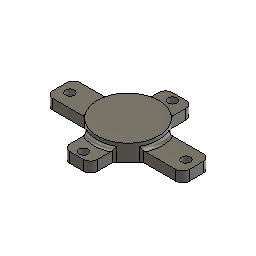
Base (Autodesk Fusion 360 design; units mm, degrees)
part number: 2025-04-16-17-35-49-953
Autodesk Fusion 360 part; units mm, degrees
sketch "Sketch1" plane through (0, 0, 0) normal (0, 1, 0) x (1, 0, 0)
  line L0 (20, 75) -> (-20, 75)
  line L1 (-100, 20) -> (-100, -20)
  line L2 (-20, -75) -> (20, -75)
  line L3 (100, -20) -> (100, 20)
  line L4 (20, 40.3113) -> (20, 75)
  line L5 (20, 75) -> (-20, 75)
  line L6 (-20, 75) -> (-20, 40.3113)
  line L7 (20, -40.3113) -> (20, -75)
  line L8 (20, -75) -> (-20, -75)
  line L9 (-20, -75) -> (-20, -40.3113)
  line L10 (40.3113, 20) -> (100, 20)
  line L11 (100, 20) -> (100, -20)
  line L12 (100, -20) -> (40.3113, -20)
  line L13 (-40.3113, 20) -> (-100, 20)
  line L14 (-100, 20) -> (-100, -20)
  line L15 (-100, -20) -> (-30, -20)
  arc A0 (-20, 40.3113) -> (-40.3113, 20) centre (0, 0) ccw
  arc A1 (40.3113, 20) -> (20, 40.3113) centre (0, 0) ccw
  arc A2 (-40.3113, -20) -> (-20, -40.3113) centre (0, 0) ccw
  arc A3 (20, -40.3113) -> (40.3113, -20) centre (0, 0) ccw
  dimension "d5" = 90
  constraint horizontal L0
  constraint perpendicular L0 L1
  constraint parallel L0 L2
  constraint parallel L1 L3
  constraint coincident A0.centre A1.centre
  constraint vertical L4
  constraint horizontal L5
  constraint vertical L6
  constraint vertical L7
  constraint horizontal L8
  constraint vertical L9
  constraint horizontal L10
  constraint vertical L11
  constraint horizontal L12
  constraint horizontal L13
  constraint vertical L14
  constraint horizontal L15
  constraint coincident L9.end A0
  constraint coincident L15 A2.start
  constraint concentric A0 A2
  constraint concentric A1 A2
  constraint coincident L7.start A2
  constraint concentric A2 A3
  measures "d5" diameter of A0
extrude "Extrude1" add sketch "Sketch1" along normal blind 15
sketch "Sketch3" plane through (0, 15, 0) normal (0, 1, 0) x (-1, 0, 0)
  line L0 (-20, 75) -> (-20, 40.3113)
  arc A0 (-20, 40.3113) -> (-40.3113, 20) centre (0, 0) ccw
  line L1 (-40.3113, 20) -> (-100, 20)
  line L2 (-100, 20) -> (-100, -20)
  line L3 (-100, -20) -> (-40.3113, -20)
  arc A1 (-40.3113, -20) -> (-20, -40.3113) centre (0, 0) ccw
  line L4 (-20, -40.3113) -> (-20, -75)
  line L5 (-20, -75) -> (20, -75)
  line L6 (20, -75) -> (20, -40.3113)
  arc A2 (20, -40.3113) -> (40.3113, -20) centre (0, 0) ccw
  line L7 (40.3113, -20) -> (100, -20)
  line L8 (100, -20) -> (100, 20)
  line L9 (100, 20) -> (40.3113, 20)
  arc A3 (40.3113, 20) -> (20, 40.3113) centre (0, 0) ccw
  line L10 (20, 40.3113) -> (20, 75)
  line L11 (20, 75) -> (-20, 75)
  circle A4 centre (0, 0) radius 45
  constraint coincident A0.centre A1.centre
extrude "Extrude2" add sketch "Sketch3" along normal blind 10 contours A0 A1 A2 A3 A4
fillet "Fillet1" radius 5 1 edges at (0, 15, 45)
fillet "Fillet2" radius 5 1 edges at (45, 15, 0)
fillet "Fillet3" radius 5 1 edges at (0, 15, -45)
fillet "Fillet4" radius 5 1 edges at (-45, 15, 0)
fillet "Fillet5" radius 5 1 edges at (-20, 10, -40.3113)
fillet "Fillet6" radius 5 1 edges at (-40.3113, 10, -20)
fillet "Fillet7" radius 5 1 edges at (-40.3113, 10, 20)
fillet "Fillet8" radius 5 1 edges at (-20, 10, 40.3113)
fillet "Fillet9" radius 5 1 edges at (20, 10, 40.3113)
fillet "Fillet10" radius 5 1 edges at (40.3113, 10, 20)
sketch "Sketch4" plane through (0, 15, 0) normal (0, 1, 0) x (-1, 0, 0)
  arc A0 (45.8258, -20) -> (45.8258, 20) centre (0, 0) ccw
  line L0 (45.8258, -20) -> (100, -20)
  line L1 (100, -20) -> (100, 20)
  line L2 (100, 20) -> (45.8258, 20)
  circle A1 centre (0, -65) radius 6.5
  circle A2 centre (0, 65) radius 6.5
  circle A3 centre (-85, 0) radius 6.5
  circle A4 centre (85, 0) radius 6.5
  dimension "d30" = 13
  dimension "d31" = 13
  dimension "d32" = 13
  dimension "d33" = 13
  measures "d30" diameter of A1
  measures "d31" diameter of A2
  measures "d32" diameter of A3
  measures "d33" diameter of A4
extrude "Extrude3" cut sketch "Sketch4" against normal blind 15 contours A1 | A2 | A3 | A4
fillet "Fillet11" radius 10 1 edges at (20, 7.5, 75)
fillet "Fillet12" radius 10 7 edges at (100, 7.5, 20) (100, 7.5, -20) (20, 7.5, -75) (-100, 7.5, 20) (-20, 7.5, 75) (-20, 7.5, -75) (-100, 7.5, -20)
sketch "Sketch5" plane through (0, 0, 0) normal (0, -1, 0) x (1, 0, 0)
  circle A0 centre (0, -65) radius 6.5
  circle A1 centre (85, 0) radius 6.5
  circle A2 centre (-85, 0) radius 6.5
  circle A3 centre (0, 65) radius 6.5
  arc A4 (-100, -10) -> (-90, -20) centre (-90, -10) ccw
  line L0 (-90, -20) -> (-43.3013, -20)
  arc A5 (-38.9711, -22.5) -> (-43.3013, -20) centre (-43.3013, -25) ccw
  arc A6 (-38.9711, -22.5) -> (-22.5, -38.9711) centre (0, 0) ccw
  arc A7 (-20, -43.3013) -> (-22.5, -38.9711) centre (-25, -43.3013) ccw
  line L1 (-20, -43.3013) -> (-20, -65)
  arc A8 (-20, -65) -> (-10, -75) centre (-10, -65) ccw
  line L2 (-10, -75) -> (10, -75)
  arc A9 (10, -75) -> (20, -65) centre (10, -65) ccw
  line L3 (20, -65) -> (20, -40.3113)
  arc A10 (20, -40.3113) -> (40.3113, -20) centre (0, 0) ccw
  line L4 (40.3113, -20) -> (90, -20)
  arc A11 (90, -20) -> (100, -10) centre (90, -10) ccw
  line L5 (100, -10) -> (100, 10)
  arc A12 (100, 10) -> (90, 20) centre (90, 10) ccw
  line L6 (90, 20) -> (43.3013, 20)
  arc A13 (38.9711, 22.5) -> (43.3013, 20) centre (43.3013, 25) ccw
  arc A14 (38.9711, 22.5) -> (22.5, 38.9711) centre (0, 0) ccw
  arc A15 (20, 43.3013) -> (22.5, 38.9711) centre (25, 43.3013) ccw
  line L7 (20, 43.3013) -> (20, 65)
  arc A16 (20, 65) -> (10, 75) centre (10, 65) ccw
  line L8 (10, 75) -> (-10, 75)
  arc A17 (-10, 75) -> (-20, 65) centre (-10, 65) ccw
  line L9 (-20, 65) -> (-20, 43.3013)
  arc A18 (-22.5, 38.9711) -> (-20, 43.3013) centre (-25, 43.3013) ccw
  arc A19 (-22.5, 38.9711) -> (-38.9711, 22.5) centre (0, 0) ccw
  arc A20 (-43.3013, 20) -> (-38.9711, 22.5) centre (-43.3013, 25) ccw
  line L10 (-43.3013, 20) -> (-90, 20)
  arc A21 (-90, 20) -> (-100, 10) centre (-90, 10) ccw
  line L11 (-100, 10) -> (-100, -10)
  circle A22 centre (0, 0) radius 25
  constraint coincident A6.centre A10.centre
extrude "Extrude4" cut sketch "Sketch5" against normal blind 10 contours A22
fillet "Fillet13" radius 5 1 edges at (-23.3082, 0, 9.0404)
